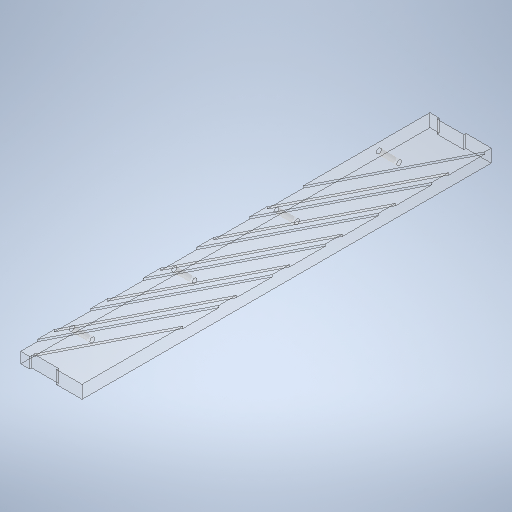
# Autodesk Inventor part: Module Cradle Right V1
Saved by Autodesk Inventor 2025 (Build 290162000, 162)
## iProperties
Created: 2024-03-20
Part Number: Module Cradle Right V1
Material: PMMA Plastic
Document SubType Name: Modeling
Designer: cfang
Density: 1.188 g/cm^3
Appearance: Polycarbonate - Clear
Author: cfang
Autodesk Inventor part; units mm, degrees
ref_plane "YZ Plane" through (0, 0, 0) normal (1, 0, 0) x (0, 1, 0)
ref_plane "XZ Plane" through (0, 0, 0) normal (0, 1, 0) x (-1, 0, 0)
ref_plane "XY Plane" through (0, 0, 0) normal (0, 0, 1) x (1, 0, 0)
sketch "Sketch3" plane through (0, 0, 0) normal (0, 1, 0) x (-1, 0, 0)
  line L0 (-15, -100) -> (15, -100)
  line L1 (15, -100) -> (15, 100)
  line L2 (15, 100) -> (-15, 100)
  line L3 (-15, 100) -> (-15, -100)
  line L4 (-15, -100) -> (15, 100) construction
  line L5 (15, -100) -> (-15, 100) construction
  point P0 (0, 0)
  dimension "d7" = 30
  dimension "d8" = 200
  constraints: 12 end point, 2 midpoint, 2 parallel, 1 horizontal, 1 perpendicular
  measures "d7" distance of L1.end L2.end
  measures "d8" distance of L0.end L1.end
extrude "Extrusion2" add sketch "Sketch3" along normal blind 6.35
sketch "Sketch5" plane through (0, 6.35, 0) normal (0, 1, 0) x (1, 0, 0)
  line L0 (-15, 100) -> (-15, -100) projected
  line L1 (-15, -109.6215) -> (15, -50.7432)
  line L2 (15, -100) -> (15, 100) projected
  line L3 (-15, -92) -> (15, -33.1217)
  line L4 (-15, -100) -> (15, -100) projected
  line L5 (-15, -66) -> (15, -7.1217)
  line L6 (-15, -83.6215) -> (15, -24.7432)
  line L7 (-15, -40) -> (15, 18.8783)
  line L8 (-15, -57.6215) -> (15, 1.2568)
  line L9 (-15, -14) -> (15, 44.8783)
  line L10 (-15, -31.6215) -> (15, 27.2568)
  line L11 (-15, 12) -> (15, 70.8783)
  line L12 (-15, -5.6215) -> (15, 53.2568)
  line L13 (-15, 38) -> (15, 96.8783)
  line L14 (-15, 20.3785) -> (15, 79.2568)
  point P0 (0, 0)
  point P1 (-10.0976, -100)
  point P2 (-15, 20.3785)
  point P3 (15, 79.2568)
  point P4 (-15, 38)
  point P5 (-15, -5.6215)
  point P6 (15, 53.2568)
  point P7 (-15, 12)
  point P8 (-15, -31.6215)
  point P9 (15, 27.2568)
  point P10 (-15, -14)
  point P11 (-15, -57.6215)
  point P12 (15, 1.2568)
  point P13 (-15, -40)
  point P14 (-15, -83.6215)
  point P15 (15, -24.7432)
  point P16 (15, -7.1217)
  point P17 (-15, -66)
  dimension "d23" = 27
  dimension "d25" = 8
  dimension "d35" = 8
  dimension "d38" = 26
  constraints: 24 end point, 4 point on line, 1 parallel, 1 vertical, 30 other
  measures "d23" angle of L0 L1
  measures "d25" distance between parallel lines of L1 L3
  measures "d35" distance from line of L4 L3.start
  measures "d38" distance of L3.start L5.start
extrude "Extrusion4" cut sketch "Sketch5" against normal blind 1 contours L13 L2 L14 L0 | L11 L2 L12 L0 | L9 L2 L10 L0 | L7 L2 L8 L0 | L5 L2 L6 L0 | L3 L2 L1 L4 L0
sketch "Sketch7" plane through (-15, 0, 100) normal (0, 0, 1) x (1, 0, 0)
  line L0 (30, 6.35) -> (0, 6.35) projected
  line L1 (4.5, 0) -> (17.5, 0)
  line L2 (17.5, 0) -> (17.5, 6.35)
  line L3 (17.5, 6.35) -> (4.5, 6.35)
  line L4 (4.5, 6.35) -> (4.5, 0)
  line L5 (0, 0) -> (0, 5.35) projected
  line L6 (0, 0) -> (30, 0) projected
  point P0 (15, 0)
  point P1 (4.5, 3.175)
  point P2 (4.5, 6.35)
  dimension "d49" = 4.5
  dimension "d50" = 17.5
  constraints: 8 end point, 2 parallel, 2 point on line, 1 horizontal, 1 midpoint, 1 perpendicular
  measures "d49" distance from line of point (4.5, 3.175) L5
  measures "d50" distance between parallel lines of L2 L5
extrude "Extrusion6" cut sketch "Sketch7" against normal blind 1
sketch "Sketch8" plane through (15, 0, -100) normal (0, 0, -1) x (-1, 0, 0)
  line L0 (0, 0) -> (30, 0) projected
  line L1 (25.5, 6.35) -> (12.5, 6.35)
  line L2 (12.5, 6.35) -> (12.5, 0)
  line L3 (12.5, 0) -> (25.5, 0)
  line L4 (25.5, 0) -> (25.5, 6.35)
  line L5 (30, 0) -> (30, 6.35) projected
  line L6 (0, 6.35) -> (30, 6.35) projected
  point P0 (15, 0)
  dimension "d53" = 4.5
  dimension "d54" = 17.5
  constraints: 8 end point, 2 parallel, 2 point on line, 1 horizontal, 1 perpendicular
  measures "d53" distance between parallel lines of L4 L5
  measures "d54" distance between parallel lines of L2 L5
extrude "Extrusion7" cut sketch "Sketch8" against normal blind 1 contours L2 L1 L4 L0
sketch "Sketch9" plane through (-15, 0, -100) normal (-1, 0, 0) x (0, 0, 1)
  line L0 (0, 0) -> (200, 0) projected
  point P0 (100, 0)
  point P1 (125, 2.675)
  point P2 (75, 2.675)
  point P3 (25, 2.675)
  point P4 (175, 2.675)
  point P5 (100, 0)
  point P6 (100, 0)
  dimension "d57" = 2.675
  dimension "d58" = 25
  dimension "d59" = 50
  dimension "d60" = 25
  dimension "d61" = 50
  constraints: 3 horizontal alignment, 2 midpoint
  measures "d57" distance from line of L0 point (25, 2.675)
  measures "d58" horizontal distance of point (75, 2.675) point (100, 0)
  measures "d59" distance of point (25, 2.675) point (75, 2.675)
  measures "d60" horizontal distance of point (100, 0) point (125, 2.675)
  measures "d61" distance of point (125, 2.675) point (175, 2.675)
hole "Hole1" at (-15, 2.675, 25) at (-15, 2.675, -25) at (-15, 2.675, -75) at (-15, 2.675, 75) direction (1, 0, 0) diameter 2.459 depth 10 tip angle 118 thread size "M3x0.5" class "6H" standard "ANSI Metric M Profile"
equation "\"d59\" = 2 * d58"
equation "\"d60\" = d58"
equation "\"d61\" = d59"
body "Solid2"
